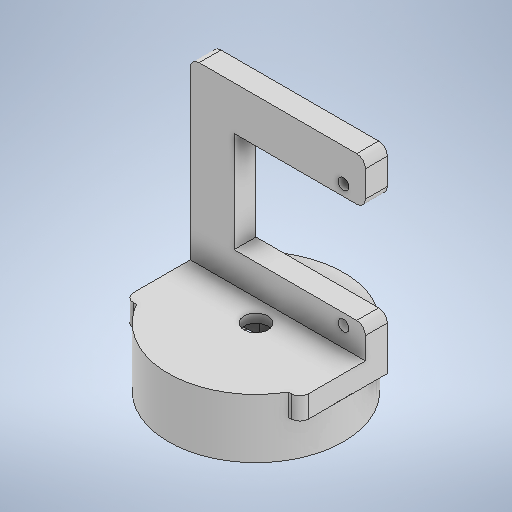
# Autodesk Inventor part: head_bottom
Saved by Autodesk Inventor 2026.1 (Build 301233000, 233)
## iProperties
Created: 2026-01-12
Part Number: head_bottom
Material: Generic
Document SubType Name: Modeling
Designer: chris
Density: 1 g/cm^3
Appearance: Default
Author: chris
Autodesk Inventor part; units mm, degrees
ref_plane "YZ Plane" through (0, 0, 0) normal (1, 0, 0) x (0, 1, 0)
ref_plane "XZ Plane" through (0, 0, 0) normal (0, 1, 0) x (-1, 0, 0)
ref_plane "XY Plane" through (0, 0, 0) normal (0, 0, 1) x (1, 0, 0)
sketch "Sketch1" plane through (0, 0, 0) normal (0, 1, 0) x (-1, 0, 0)
  line L0 (-20, 20) -> (20, 20)
  line L1 (20, 20) -> (20, -20)
  line L2 (20, -20) -> (-20, -20)
  line L3 (-20, -20) -> (-20, 20)
  line L4 (-20, 20) -> (20, -20) construction
  line L5 (20, 20) -> (-20, -20) construction
  point P0 (0, 0)
  dimension "d0" = 40
  dimension "d1" = 40
  constraints: 12 end point, 2 midpoint, 2 parallel, 1 horizontal, 1 perpendicular
  measures "d0" distance of L1.end L2.end
  measures "d1" distance of L0.end L1.end
extrude "Extrusion1" add sketch "Sketch1" along normal blind 5
sketch "Sketch4" plane through (0, 5, 0) normal (0, 1, 0) x (1, 0, 0)
  line L0 (-20, 10) -> (-10, 10)
  line L1 (-10, 10) -> (-10, 5)
  line L2 (-10, 5) -> (-20, 5)
  line L3 (-20, 5) -> (-20, 10)
  line L4 (-20, 10) -> (-10, 5) construction
  line L5 (-10, 10) -> (-20, 5) construction
  line L6 (-20, -20) -> (20, -20) projected
  line L7 (20, -20) -> (20, 20) projected
  line L8 (-20, 20) -> (-20, -20) projected
  point P0 (-15, 7.5)
  dimension "d20" = 10
  dimension "d21" = 5
  dimension "d23" = 25
  constraints: 12 end point, 2 midpoint, 2 parallel, 1 collinear, 1 horizontal, 1 perpendicular
  measures "d20" distance of L1.end L2.end
  measures "d21" distance of L0.end L1.end
  measures "d23" distance between parallel lines of L6 L2
extrude "Extrusion4" add sketch "Sketch4" along normal blind 40
sketch "Sketch8" plane through (-10, 5, -5) normal (1, 0, 0) x (0, 0, -1)
  line L0 (0, 40) -> (5, 40)
  line L1 (5, 40) -> (5, 30)
  line L2 (5, 30) -> (0, 30)
  line L3 (0, 30) -> (0, 40)
  line L4 (0, 7) -> (5, 7)
  line L5 (5, 7) -> (5, 0)
  line L6 (5, 0) -> (0, 0)
  line L7 (0, 0) -> (0, 7)
  line L8 (5, 0) -> (5, 40) projected
  line L9 (0, 40) -> (5, 40) projected
  point P0 (-5, -5)
  dimension "d44" = 5
  dimension "d45" = 10
  dimension "d46" = 5
  dimension "d47" = 7
  dimension "d48" = 23
  constraints: 16 end point, 4 parallel, 3 collinear, 2 horizontal, 2 perpendicular
  measures "d44" distance of L1.end L2.end
  measures "d45" distance of L2.end L0.start
  measures "d46" distance of L5.end L6.end
  measures "d47" distance of L6.end L4.start
  measures "d48" distance between parallel lines of L4 L2
extrude "Extrusion7" add sketch "Sketch8" along normal blind 30
sketch "Sketch9" plane through (-20, 5, -5) normal (0, 0, 1) x (1, 0, 0)
  circle A0 centre (35, 32.5) radius 1.25
  circle A1 centre (35, 4.5) radius 1.25
  line L0 (10, 30) -> (40, 30) projected
  line L1 (40, 40) -> (40, 30) projected
  line L2 (40, 7) -> (40, 0) projected
  point P0 (20, -5)
  dimension "d51" = 2.5
  dimension "d52" = 2.5
  dimension "d53" = 28
  dimension "d54" = 2.5
  dimension "d55" = 5
  dimension "d56" = 5
  constraints: 2 centre point
  measures "d51" diameter of A0
  measures "d52" diameter of A1
  measures "d53" distance of A1.centre A0.centre
  measures "d54" distance from line of L0 A0.centre
  measures "d55" distance from line of L1 A0.centre
  measures "d56" distance from line of L2 A1.centre
extrude "Extrusion8" cut sketch "Sketch9" against normal blind 5
sketch "Sketch11" plane through (0, 5, 0) normal (0, 1, 0) x (1, 0, 0)
  line L0 (20, -20) -> (-20, -20)
  line L1 (-20, -20) -> (-20, -10)
  line L2 (-20, -10) -> (20, -10)
  line L3 (20, -10) -> (20, -20)
  line L4 (-20, 10) -> (20, 10)
  line L5 (20, 10) -> (20, 20)
  line L6 (20, 20) -> (-20, 20)
  line L7 (-20, 20) -> (-20, 10)
  line L8 (20, 20) -> (-20, 20) projected
  line L9 (-20, -20) -> (20, -20) projected
  line L10 (20, -20) -> (20, 5) projected
  line L11 (20, 10) -> (20, 20) projected
  point P0 (0, 0)
  dimension "d59" = 40
  dimension "d60" = 10
  dimension "d61" = 40
  dimension "d62" = 10
  constraints: 16 end point, 4 collinear, 4 parallel, 2 horizontal, 2 perpendicular
  measures "d59" distance of L1.end L2.end
  measures "d60" distance of L0.end L1.end
  measures "d61" distance of L6.end L5.end
  measures "d62" distance of L5.end L4.end
extrude "Extrusion9" cut sketch "Sketch11" against normal blind 5
sketch "Sketch12" plane through (0, 0, 0) normal (0, -1, 0) x (1, 0, 0)
  circle A0 centre (0, 0) radius 3.5
  circle A1 centre (14, 0) radius 2.5
  circle A2 centre (-14, 0) radius 2.5
  line L0 (-20, -10) -> (20, -10) projected
  line L1 (-14, 2.5) -> (-2.0057, 2.8683)
  line L2 (-14, -2.5) -> (-2.0057, -2.8683)
  line L3 (14, 2.5) -> (2.0057, 2.8683)
  line L4 (14, -2.5) -> (2.0057, -2.8683)
  dimension "d65" = 7
  dimension "d66" = 5
  dimension "d67" = 5
  dimension "d68" = 14
  dimension "d69" = 10
  dimension "d70" = 10
  dimension "d71" = 14
  dimension "d72" = 12
  dimension "d73" = 12
  constraints: 8 end point, 8 point on circle, 3 centre point, 1 coincident, 1 parallel
  measures "d65" diameter of A0
  measures "d66" diameter of A1
  measures "d67" diameter of A2
  measures "d68" distance of A1.centre point (0, 0)
  measures "d69" distance from line of L0 A1.centre
  measures "d70" distance from line of L0 A2.centre
  measures "d71" distance of A2.centre point (0, 0)
  measures "d72" distance of L1.start L1.end
  measures "d73" distance of L4.start L4.end
extrude "Extrusion10" cut sketch "Sketch12" against normal blind 3
sketch "Sketch13" plane through (0, 3, 0) normal (0, -1, 0) x (1, 0, 0)
  circle A0 centre (0, 0) radius 2.75
  dimension "d76" = 5.5
  constraints: 1 centre point, 1 coincident
  measures "d76" diameter of A0
extrude "Extrusion11" cut sketch "Sketch13" against normal blind 3
fillet "Fillet1" radius 2 6 edges at (20, 45, -7.5) (20, 35, -7.5) (20, 12, -7.5) (20, 2.5, 10) (-20, 2.5, 10) (-20, 45, -7.5)
sketch "Sketch14" plane through (0, 0, 0) normal (0, -1, 0) x (1, 0, 0)
  circle A0 centre (0, 0) radius 17.5
  circle A1 centre (0, 0) radius 20
  dimension "d80" = 35
  dimension "d81" = 40
  constraints: 2 centre point, 2 coincident
  measures "d80" diameter of A0
  measures "d81" diameter of A1
extrude "Extrusion12" add sketch "Sketch14" along normal blind 8.5
sketch "Sketch15" plane through (0, 0, 0) normal (0, -1, 0) x (1, 0, 0)
  circle A0 centre (0, 0) radius 17.5 projected
  arc A1 (2.0057, 2.8683) -> (-2.0057, 2.8683) centre (0, 0) ccw projected
  line L0 (2.0057, 2.8683) -> (14, 2.5) projected
  arc A2 (14, -2.5) -> (14, 2.5) centre (14, 0) ccw projected
  line L1 (14, -2.5) -> (2.0057, -2.8683) projected
  arc A3 (-2.0057, -2.8683) -> (2.0057, -2.8683) centre (0, 0) ccw projected
  line L2 (-2.0057, -2.8683) -> (-14, -2.5) projected
  arc A4 (-14, 2.5) -> (-14, -2.5) centre (-14, 0) ccw projected
  line L3 (-14, 2.5) -> (-2.0057, 2.8683) projected
  arc A5 (14.3614, -10) -> (14.3614, 10) centre (0, 0) ccw projected
  line L4 (14.3614, 10) -> (-14.3614, 10) projected
  arc A6 (-14.3614, 10) -> (-14.3614, -10) centre (0, 0) ccw projected
  line L5 (-14.3614, -10) -> (14.3614, -10) projected
  circle A7 centre (0, 0) radius 20 projected
  point P0 (14.3614, 10)
extrude "Extrusion13" add sketch "Sketch15" against normal blind 5 contours L4 A0 | A0 L5 | A7
body "Solid1"
